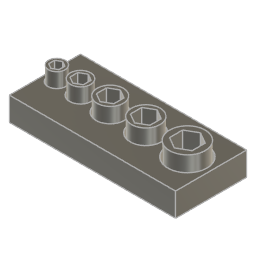
0 (Autodesk Fusion 360 design; units mm, degrees)
part number: 2026-08-15-12-15-00-669
Autodesk Fusion 360 part; units mm, degrees
note: some values were not read from the file. Chosen so that the rebuilt part matches the saved one: which bodies a step acts on. Set by a fixed rule: which sketch regions a step uses.
sketch "Skizze1" plane through (0, 0, 0) normal (0, 0, 1) x (1, 0, 0)
  line L0 (0, 0) -> (140, 0)
  line L1 (140, 0) -> (140, 60)
  line L2 (140, 60) -> (0, 60)
  line L3 (0, 60) -> (0, 0)
  dimension "d26" = 140
  dimension "d27" = 60
  constraint horizontal L0
  constraint vertical L1
  constraint horizontal L2
  constraint vertical L3
  constraint coincident L0.start L3.end
  measures "d26" distance of L1 L3
  measures "d27" distance of L0 L2
extrude "Extrusion1" add sketch "Skizze1" along normal blind 20 makes body 1
sketch "Skizze2" plane through (0, 0, 20) normal (0, 0, 1) x (-1, 0, 0)
  line L0 (0, -60) -> (0, 0)
  line L1 (0, 0) -> (-140, 0)
  line L2 (-140, 0) -> (-140, -60)
  line L3 (-140, -60) -> (0, -60)
  line L4 (0, -30) -> (-140, -30)
  circle A0 centre (-10, -30) radius 7.5
  circle A1 centre (-30, -30) radius 9.25
  circle A2 centre (-55, -30) radius 12
  circle A3 centre (-85, -30) radius 13.25
  circle A4 centre (-120, -30) radius 16.5
  line L5 (0, -60) -> (0, 0)
  dimension "d4" = 15
  dimension "d5" = 18.5
  dimension "d6" = 24
  dimension "d7" = 26.5
  dimension "d28" = 33
  dimension "d29" = 20
  dimension "d30" = 25
  dimension "d31" = 30
  dimension "d32" = 35
  dimension "d33" = 10
  constraint midpoint L0 L4.start
  constraint midpoint L2 L4.end
  constraint coincident L4 A0.centre
  constraint coincident L4 A1.centre
  constraint coincident L4 A2.centre
  constraint coincident L4 A3.centre
  constraint coincident L4 A4.centre
  measures "d4" diameter of A0
  measures "d5" diameter of A1
  measures "d6" diameter of A2
  measures "d7" diameter of A3
  measures "d28" diameter of A4
  measures "d29" distance of A0.centre A1.centre
  measures "d30" distance of A1.centre A2.centre
  measures "d31" distance of A2.centre A3.centre
  measures "d32" distance of A3.centre A4.centre
  measures "d33" distance of A0.centre L5
sketch "Skizze3" plane through (0, 0, 20) normal (0, 0, 1) x (-1, 0, 0)
  line L0 (0, -30) -> (-140, -30)
  line L1 (-34.75, -34.75) -> (-25.25, -34.75)
  line L2 (-25.25, -34.75) -> (-25.25, -25.25)
  line L3 (-25.25, -25.25) -> (-34.75, -25.25)
  line L4 (-34.75, -25.25) -> (-34.75, -34.75)
  line L5 (-14.75, -25.25) -> (-14.75, -34.75)
  line L6 (-14.75, -34.75) -> (-5.25, -34.75)
  line L7 (-5.25, -34.75) -> (-5.25, -25.25)
  line L8 (-5.25, -25.25) -> (-14.75, -25.25)
  line L9 (-30, -39) -> (-30, -21)
  line L10 (-55, -42) -> (-55, -18)
  line L11 (-85, -43) -> (-85, -17) construction
  line L12 (-120.0777, -46.4998) -> (-120.0777, -13.5002) construction
  line L13 (-50.25, -34.75) -> (-59.75, -34.75)
  line L14 (-59.75, -34.75) -> (-59.75, -25.25)
  line L15 (-59.75, -25.25) -> (-50.25, -25.25)
  line L16 (-50.25, -25.25) -> (-50.25, -34.75)
  line L17 (-80.25, -34.75) -> (-89.75, -34.75)
  line L18 (-89.75, -34.75) -> (-89.75, -25.25)
  line L19 (-89.75, -25.25) -> (-80.25, -25.25)
  line L20 (-80.25, -25.25) -> (-80.25, -34.75)
  line L21 (-115.25, -34.75) -> (-124.75, -34.75)
  line L22 (-124.75, -34.75) -> (-124.75, -25.25)
  line L23 (-124.75, -25.25) -> (-115.25, -25.25)
  line L24 (-115.25, -25.25) -> (-115.25, -34.75)
  line L25 (-10, -37.5) -> (-10, -22.5213)
  line L26 (0, -60) -> (0, 0)
  line L27 (0, 0) -> (-140, 0)
  line L28 (-140, 0) -> (-140, -60)
  line L29 (-140, -60) -> (0, -60)
  point P0 (-10, -30)
  point P1 (-30, -30)
  point P2 (-55, -30)
  point P3 (-85, -30)
  point P4 (-120, -30)
  dimension "d14" = 9.5
  dimension "d15" = 9.5
  dimension "d16" = 9.5
  dimension "d17" = 9.5
  dimension "d34" = 9.5
  dimension "d35" = 9.5
  dimension "d36" = 9.5
  dimension "d37" = 9.5
  dimension "d38" = 9.5
  dimension "d39" = 9.5
  dimension "d40" = 4.75
  dimension "d41" = 4.75
  dimension "d42" = 4.75
  dimension "d43" = 4.75
  dimension "d44" = 4.75
  dimension "d45" = 4.75
  dimension "d46" = 4.75
  dimension "d47" = 4.75
  dimension "d48" = 4.75
  dimension "d49" = 4.75
  constraint horizontal L1
  constraint vertical L2
  constraint horizontal L3
  constraint vertical L4
  constraint horizontal L6
  constraint vertical L7
  constraint horizontal L8
  constraint vertical L5
  constraint parallel L2 L9
  constraint vertical L10
  constraint perpendicular L0 L11
  constraint vertical L12
  constraint horizontal L13
  constraint vertical L14
  constraint horizontal L15
  constraint vertical L16
  constraint horizontal L17
  constraint vertical L18
  constraint horizontal L19
  constraint vertical L20
  constraint horizontal L21
  constraint vertical L22
  constraint horizontal L23
  constraint vertical L24
  constraint perpendicular L6 L25
  measures "d14" distance of L2.end L3.end
  measures "d15" distance of L1.end L2.end
  measures "d16" distance of L5.start L7.end
  measures "d17" distance of L7.end L6.end
  measures "d34" distance of L13.start L15.end
  measures "d35" distance of L14 L16
  measures "d36" distance of L17.start L19.end
  measures "d37" distance of L18 L20
  measures "d38" distance of L21.start L23.end
  measures "d39" distance of L22 L24
  measures "d40" distance of L5 P0
  measures "d41" distance of L8 P0
  measures "d42" distance of L4 P1
  measures "d43" distance of L3 P1
  measures "d44" distance of L15 P2
  measures "d45" distance of L14 P2
  measures "d46" distance of L18 P3
  measures "d47" distance of L19 P3
  measures "d48" distance of L23 P4
  measures "d49" distance of L22 P4
extrude "Extrusion3" cut sketch "Skizze2" against normal blind 12 contours L4 A0 | L4 A0 | L4 A4 | L4 A4 | L4 A1 | L4 A1 | L4 A3 | L4 A3 | L4 A2 | L4 A2 bodies 1
extrude "Extrusion4" add sketch "Skizze3" along normal blind 7 from surface at -12 contours L0 L6 L7 L25 | L0 L7 L8 L25 | L0 L5 L6 L25 | L0 L5 L8 L25 | L0 L1 L2 L9 | L0 L2 L3 L9 | L0 L22 L23 L24 | L0 L21 L22 L24 | L0 L1 L4 L9 | L0 L3 L4 L9 | L0 L18 L19 L20 | L0 L17 L18 L20 | L0 L10 L13 L16 | L0 L10 L15 L16 | L0 L10 L13 L14 | L0 L10 L14 L15 bodies 1
fillet "Abrundung1" radius 2 20 edges at (14.75, 30, 15) (10, 34.75, 15) (5.25, 30, 15) (10, 25.25, 15) (30, 34.75, 15) (25.25, 30, 15) (30, 25.25, 15) (34.75, 30, 15) (50.25, 30, 15) (55, 34.75, 15) (55, 25.25, 15) (59.75, 30, 15) (80.25, 30, 15) (85, 34.75, 15) (89.75, 30, 15) (85, 25.25, 15) (115.25, 30, 15) (120, 34.75, 15) (124.75, 30, 15) (120, 25.25, 15) on bodies 1
sketch "Skizze4" plane through (0, 0, 20) normal (0, 0, 1) x (-1, 0, 0)
  circle A0 centre (-10, -30) radius 7
  circle A1 centre (-30, -30) radius 8.5
  circle A2 centre (-55, -30) radius 11
  circle A3 centre (-55, -30) radius 12
  circle A4 centre (-85, -30) radius 12
  circle A5 centre (-120, -30) radius 15
  circle A6 centre (-120, -30) radius 16.5
  circle A7 centre (-85, -30) radius 13.25
  circle A8 centre (-10, -30) radius 7.5
  circle A9 centre (-30, -30) radius 9.25
  circle A10 centre (-55, -30) radius 12
  dimension "d57" = 14
  dimension "d58" = 33
  dimension "d59" = 26.5
  dimension "d60" = 15
  dimension "d61" = 18.5
  dimension "d62" = 24
  dimension "d63" = 14
  dimension "d64" = 17
  dimension "d65" = 22
  dimension "d66" = 24
  dimension "d67" = 30
  constraint concentric A2 A3
  measures "d57" diameter of A0
  measures "d58" diameter of A6
  measures "d59" diameter of A7
  measures "d60" diameter of A8
  measures "d61" diameter of A9
  measures "d62" diameter of A10
  measures "d63" diameter of A0
  measures "d64" diameter of A1
  measures "d65" diameter of A2
  measures "d66" diameter of A4
  measures "d67" diameter of A5
extrude "Extrusion5" add sketch "Skizze4" along normal mid plane 24 separate body contours A0 | A1 | A2 | A4 | A5 makes body 2 at (44.0137, 30.5483, 28) makes body 3 at (73.0149, 30.5981, 28) makes body 4 at (21.5106, 30.4237, 28) makes body 5 at (105.0186, 30.7477, 28) makes body 6 at (3.0087, 30.3489, 28)
sketch "Skizze5" plane through (0, 0, 8) normal (0, 0, -1) x (1, 0, 0)
  circle A0 centre (30, -30) radius 8.5
  line L0 (0, -30) -> (140, -30)
  line L1 (25.25, -25.25) -> (34.75, -25.25)
  line L2 (34.75, -25.25) -> (34.75, -34.75)
  line L3 (34.75, -34.75) -> (25.25, -34.75)
  line L4 (25.25, -34.75) -> (25.25, -25.25)
  line L5 (50.25, -25.25) -> (59.75, -25.25)
  line L6 (59.75, -25.25) -> (59.75, -34.75)
  line L7 (59.75, -34.75) -> (50.25, -34.75)
  line L8 (50.25, -34.75) -> (50.25, -25.25)
  line L9 (80.25, -25.25) -> (89.75, -25.25)
  line L10 (89.75, -25.25) -> (89.75, -34.75)
  line L11 (89.75, -34.75) -> (80.25, -34.75)
  line L12 (80.25, -34.75) -> (80.25, -25.25)
  line L13 (115.25, -25.25) -> (124.75, -25.25)
  line L14 (124.75, -25.25) -> (124.75, -34.75)
  line L15 (124.75, -34.75) -> (115.25, -34.75)
  line L16 (115.25, -34.75) -> (115.25, -25.25)
  line L17 (10, -23) -> (10, -37)
  line L18 (30, -21.5) -> (30, -38.5)
  line L19 (55, -19) -> (55, -41)
  line L20 (85, -18) -> (85, -42)
  line L21 (120, -15) -> (120, -45)
  line L22 (0, 0) -> (140, 0)
  line L23 (140, -60) -> (0, -60)
  line L24 (5.25, -25.25) -> (14.75, -25.25)
  line L25 (14.75, -25.25) -> (14.75, -34.75)
  line L26 (14.75, -34.75) -> (5.25, -34.75)
  line L27 (5.25, -34.75) -> (5.25, -25.25)
  point P0 (120, -30)
  point P1 (85, -30)
  point P2 (55, -30)
  point P3 (30, -30)
  point P4 (10, -30)
  dimension "d72" = 9.5
  dimension "d73" = 9.5
  dimension "d74" = 9.5
  dimension "d75" = 9.5
  dimension "d76" = 9.5
  dimension "d77" = 9.5
  dimension "d78" = 9.5
  dimension "d79" = 9.5
  dimension "d81" = 4.75
  dimension "d82" = 4.75
  dimension "d83" = 4.75
  dimension "d84" = 4.75
  dimension "d85" = 4.75
  dimension "d86" = 4.75
  dimension "d87" = 4.75
  dimension "d88" = 4.75
  dimension "d89" = 9.5
  dimension "d90" = 9.5
  dimension "d91" = 4.75
  dimension "d92" = 4.75
  constraint horizontal L0
  constraint horizontal L1
  constraint vertical L2
  constraint horizontal L3
  constraint vertical L4
  constraint horizontal L5
  constraint vertical L6
  constraint horizontal L7
  constraint vertical L8
  constraint horizontal L9
  constraint vertical L10
  constraint horizontal L11
  constraint vertical L12
  constraint horizontal L13
  constraint vertical L14
  constraint horizontal L15
  constraint vertical L16
  constraint vertical L17
  constraint coincident A0 L18.start
  constraint coincident A0 L18.end
  constraint perpendicular L0 L18
  constraint perpendicular L7 L19
  constraint perpendicular L9 L20
  constraint perpendicular L13 L21
  constraint symmetric L0 L22 L23
  constraint horizontal L24
  constraint vertical L25
  constraint horizontal L26
  constraint vertical L27
  measures "d72" distance of L1.start L3.end
  measures "d73" distance of L2 L4
  measures "d74" distance of L5.start L7.end
  measures "d75" distance of L6 L8
  measures "d76" distance of L9.start L11.end
  measures "d77" distance of L10 L12
  measures "d78" distance of L13.start L15.end
  measures "d79" distance of L14 L16
  measures "d81" distance of L14 P0
  measures "d82" distance of L13 P0
  measures "d83" distance of L11 P1
  measures "d84" distance of L10 P1
  measures "d85" distance of L6 P2
  measures "d86" distance of L7 P2
  measures "d87" distance of L3 P3
  measures "d88" distance of L2 P3
  measures "d89" distance of L24.start L26.end
  measures "d90" distance of L25 L27
  measures "d91" distance of L25 P4
  measures "d92" distance of L24 P4
extrude "Extrusion6" cut sketch "Skizze5" against normal blind 7 contours L0 L2 L3 L18 | L0 L1 L2 L18 | L0 L1 L4 L18 | L0 L3 L4 L18 | L0 L17 L24 L27 | L0 L17 L26 L27 | L0 L17 L24 L25 | L0 L17 L25 L26 | L0 L5 L8 L19 | L0 L7 L8 L19 | L0 L5 L6 L19 | L0 L6 L7 L19 | L0 L9 L12 L20 | L0 L11 L12 L20 | L0 L9 L10 L20 | L0 L10 L11 L20 | L0 L13 L16 L21 | L0 L15 L16 L21 | L0 L13 L14 L21 | L0 L14 L15 L21 bodies 2 3 4 5 6
fillet "Abrundung2" radius 0.3 4 edges at (14.75, 30, 8) (10, 25.25, 8) (5.25, 30, 8) (10, 34.75, 8) on bodies 6
fillet "Abrundung3" radius 1 4 edges at (25.25, 30, 8) (30, 25.25, 8) (30, 34.75, 8) (34.75, 30, 8) on bodies 4
fillet "Abrundung4" radius 2 12 edges at (50.25, 30, 8) (55, 25.25, 8) (55, 34.75, 8) (59.75, 30, 8) (80.25, 30, 8) (85, 25.25, 8) (85, 34.75, 8) (89.75, 30, 8) (115.25, 30, 8) (120, 25.25, 8) (124.75, 30, 8) (120, 34.75, 8) on bodies 2 3 5
sketch "Skizze6" plane through (0, 0, 32) normal (0, 0, 1) x (-1, 0, 0)
  circle A0 centre (-120, -30) radius 15
  line L0 (0, -30) -> (-140, -30)
  circle A1 centre (-10, -30) radius 7
  circle A2 centre (-30, -30) radius 8.5
  circle A3 centre (-55, -30) radius 11
  circle A4 centre (-85, -30) radius 12
  line L1 (-10, -35) -> (-5.6699, -32.5)
  line L2 (-5.6699, -32.5) -> (-5.6699, -27.5)
  line L3 (-5.6699, -27.5) -> (-10, -25)
  line L4 (-10, -25) -> (-14.3301, -27.5)
  line L5 (-14.3301, -27.5) -> (-14.3301, -32.5)
  line L6 (-14.3301, -32.5) -> (-10, -35)
  line L7 (-30, -36.5) -> (-24.3708, -33.25)
  line L8 (-24.3708, -33.25) -> (-24.3708, -26.75)
  line L9 (-24.3708, -26.75) -> (-30, -23.5)
  line L10 (-30, -23.5) -> (-35.6292, -26.75)
  line L11 (-35.6292, -26.75) -> (-35.6292, -33.25)
  line L12 (-35.6292, -33.25) -> (-30, -36.5)
  line L13 (-55, -38.5) -> (-47.6388, -34.25)
  line L14 (-47.6388, -34.25) -> (-47.6388, -25.75)
  line L15 (-47.6388, -25.75) -> (-55, -21.5)
  line L16 (-55, -21.5) -> (-62.3612, -25.75)
  line L17 (-62.3612, -25.75) -> (-62.3612, -34.25)
  line L18 (-62.3612, -34.25) -> (-55, -38.5)
  line L19 (-85, -39.5) -> (-76.7728, -34.75)
  line L20 (-76.7728, -34.75) -> (-76.7728, -25.25)
  line L21 (-76.7728, -25.25) -> (-85, -20.5)
  line L22 (-85, -20.5) -> (-93.2272, -25.25)
  line L23 (-93.2272, -25.25) -> (-93.2272, -34.75)
  line L24 (-93.2272, -34.75) -> (-85, -39.5)
  line L25 (-120, -41) -> (-110.4737, -35.5)
  line L26 (-110.4737, -35.5) -> (-110.4737, -24.5)
  line L27 (-110.4737, -24.5) -> (-120, -19)
  line L28 (-120, -19) -> (-129.5263, -24.5)
  line L29 (-129.5263, -24.5) -> (-129.5263, -35.5)
  line L30 (-129.5263, -35.5) -> (-120, -41)
  point P0 (-10, -30)
  point P1 (-30, -30)
  point P2 (-55, -30)
  point P3 (-85, -30)
  point P4 (-120, -30)
  dimension "d106" = 14
  dimension "d107" = 17
  dimension "d108" = 22
  dimension "d109" = 24
  dimension "d110" = 30
  dimension "d113" = 10
  dimension "d114" = 13
  dimension "d115" = 17
  dimension "d116" = 19
  dimension "d117" = 22
  constraint horizontal L0
  constraint coincident P1 A2.centre
  constraint coincident P2 A3.centre
  constraint coincident P4 A0.centre
  measures "d106" diameter of A1
  measures "d107" diameter of A2
  measures "d108" diameter of A3
  measures "d109" diameter of A4
  measures "d110" diameter of A0
  measures "d113" distance of L1.start L3.end
  measures "d114" distance of L7.start L9.end
  measures "d115" distance of L13.start L15.end
  measures "d116" distance of L19.start L21.end
  measures "d117" distance of L25.start L27.end
extrude "Extrusion8" cut sketch "Skizze6" against normal blind 14 contours L0 L25 L26 L29 L30 | L0 L26 L27 L28 L29 | L0 L1 L2 L5 L6 | L0 L2 L3 L4 L5 | L0 L7 L8 L11 L12 | L0 L8 L9 L10 L11 | L0 L13 L14 L17 L18 | L0 L14 L15 L16 L17 | L0 L19 L20 L23 L24 | L0 L20 L21 L22 L23 bodies 2 3 4 5 6
